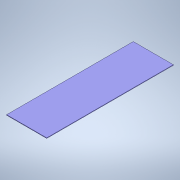
# Autodesk Inventor part: AluminumSheet
Saved by Autodesk Inventor 2021 (Build 250183000, 183)
## iProperties
Created: 2022-02-04
Part Number: AluminumSheet
Material: Generic
Document SubType Name: Modeling
Designer: tlar613
Density: 1 g/cm^3
Appearance: Default
Author: tlar613
Autodesk Inventor part; units mm, degrees
ref_plane "YZ Plane" through (0, 0, 0) normal (1, 0, 0) x (0, 1, 0)
ref_plane "XZ Plane" through (0, 0, 0) normal (0, 1, 0) x (-1, 0, 0)
ref_plane "XY Plane" through (0, 0, 0) normal (0, 0, 1) x (1, 0, 0)
sketch "Sketch1" plane through (0, 0, 0) normal (0, 1, 0) x (-1, 0, 0)
  line L0 (150, 474.1) -> (-150, 474.1)
  line L1 (-150, 474.1) -> (-150, -474.1)
  line L2 (-150, -474.1) -> (150, -474.1)
  line L3 (150, -474.1) -> (150, 474.1)
  line L4 (0, -663.74) -> (0, 663.74) projected
  line L5 (-210, 0) -> (210, 0) projected
  point P0 (0, 0)
  dimension "d0" = 948.2
  dimension "d1" = 300
  constraints: 8 end point, 2 parallel, 1 horizontal, 1 perpendicular, 2 other
  measures "d0" distance of L2.end L0.start
  measures "d1" distance of L1.end L2.end
extrude "Extrusion1" add sketch "Sketch1" along normal blind 4
body "Solid1"
